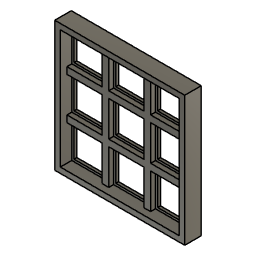
Master Assembly (Autodesk Fusion 360 archive; units mm, degrees)
design "Case Keys"
Autodesk Fusion 360 part; units mm, degrees
sketch "Sketch1" plane through (0, 0, 0) normal (0, 1, 0) x (1, 0, 0)
  line L0 (0, 0) -> (19.05, 0)
  line L1 (19.05, 0) -> (19.05, -19.05)
  line L2 (19.05, -19.05) -> (0, -19.05)
  line L3 (0, -19.05) -> (0, 0)
  line L4 (2.525, -2.525) -> (16.525, -2.525)
  line L5 (16.525, -2.525) -> (16.525, -16.525)
  line L6 (16.525, -16.525) -> (2.525, -16.525)
  line L7 (2.525, -16.525) -> (2.525, -2.525)
  line L8 (35.575, -16.525) -> (21.575, -16.525)
  line L9 (21.575, -2.525) -> (35.575, -2.525)
  line L10 (19.05, -19.05) -> (19.05, 0)
  line L11 (19.05, 0) -> (38.1, 0)
  line L12 (38.1, -19.05) -> (19.05, -19.05)
  line L13 (35.575, -2.525) -> (35.575, -16.525)
  line L14 (38.1, 0) -> (38.1, -19.05)
  line L15 (21.575, -16.525) -> (21.575, -2.525)
  line L16 (54.625, -16.525) -> (40.625, -16.525)
  line L17 (40.625, -2.525) -> (54.625, -2.525)
  line L18 (38.1, -19.05) -> (38.1, 0)
  line L19 (38.1, 0) -> (57.15, 0)
  line L20 (57.15, -19.05) -> (38.1, -19.05)
  line L21 (54.625, -2.525) -> (54.625, -16.525)
  line L22 (57.15, 0) -> (57.15, -19.05)
  line L23 (40.625, -16.525) -> (40.625, -2.525)
  line L24 (16.525, 2.525) -> (2.525, 2.525)
  line L25 (2.525, 16.525) -> (16.525, 16.525)
  line L26 (0, 0) -> (0, 19.05)
  line L27 (0, 19.05) -> (19.05, 19.05)
  line L28 (19.05, 0) -> (0, 0)
  line L29 (16.525, 16.525) -> (16.525, 2.525)
  line L30 (19.05, 19.05) -> (19.05, 0)
  line L31 (2.525, 2.525) -> (2.525, 16.525)
  line L32 (35.575, 2.525) -> (21.575, 2.525)
  line L33 (21.575, 16.525) -> (35.575, 16.525)
  line L34 (19.05, 0) -> (19.05, 19.05)
  line L35 (19.05, 19.05) -> (38.1, 19.05)
  line L36 (38.1, 0) -> (19.05, 0)
  line L37 (35.575, 16.525) -> (35.575, 2.525)
  line L38 (38.1, 19.05) -> (38.1, 0)
  line L39 (21.575, 2.525) -> (21.575, 16.525)
  line L40 (54.625, 2.525) -> (40.625, 2.525)
  line L41 (40.625, 16.525) -> (54.625, 16.525)
  line L42 (38.1, 0) -> (38.1, 19.05)
  line L43 (38.1, 19.05) -> (57.15, 19.05)
  line L44 (57.15, 0) -> (38.1, 0)
  line L45 (54.625, 16.525) -> (54.625, 2.525)
  line L46 (57.15, 19.05) -> (57.15, 0)
  line L47 (40.625, 2.525) -> (40.625, 16.525)
  line L48 (16.525, 21.575) -> (2.525, 21.575)
  line L49 (2.525, 35.575) -> (16.525, 35.575)
  line L50 (0, 19.05) -> (0, 38.1)
  line L51 (0, 38.1) -> (19.05, 38.1)
  line L52 (19.05, 19.05) -> (0, 19.05)
  line L53 (16.525, 35.575) -> (16.525, 21.575)
  line L54 (19.05, 38.1) -> (19.05, 19.05)
  line L55 (2.525, 21.575) -> (2.525, 35.575)
  line L56 (35.575, 21.575) -> (21.575, 21.575)
  line L57 (21.575, 35.575) -> (35.575, 35.575)
  line L58 (19.05, 19.05) -> (19.05, 38.1)
  line L59 (19.05, 38.1) -> (38.1, 38.1)
  line L60 (38.1, 19.05) -> (19.05, 19.05)
  line L61 (35.575, 35.575) -> (35.575, 21.575)
  line L62 (38.1, 38.1) -> (38.1, 19.05)
  line L63 (21.575, 21.575) -> (21.575, 35.575)
  line L64 (54.625, 21.575) -> (40.625, 21.575)
  line L65 (40.625, 35.575) -> (54.625, 35.575)
  line L66 (38.1, 19.05) -> (38.1, 38.1)
  line L67 (38.1, 38.1) -> (57.15, 38.1)
  line L68 (57.15, 19.05) -> (38.1, 19.05)
  line L69 (54.625, 35.575) -> (54.625, 21.575)
  line L70 (57.15, 38.1) -> (57.15, 19.05)
  line L71 (40.625, 21.575) -> (40.625, 35.575)
  circle A0 centre (9.525, -9.525) radius 1
  point P0 (19.05, 0)
  point P1 (38.1, 0)
  point P2 (0, 19.05)
  point P3 (19.05, 19.05)
  point P4 (38.1, 19.05)
  point P5 (0, 38.1)
  point P6 (19.05, 38.1)
  point P7 (38.1, 38.1)
  dimension "d13" = 19.05
  dimension "d14" = 19.05
  dimension "d15" = 2.525
  dimension "d18" = 38.1
  dimension "d19" = 38.1
  dimension "d41" = 2
  constraint horizontal L0
  constraint vertical L1
  constraint horizontal L2
  constraint vertical L3
  constraint coincident L0.start L3.end
  measures "d13" distance of L0.start L2.end
  measures "d14" distance of L0.start P0
  measures "d41" diameter of A0
extrude "Extrude1" add sketch "Sketch1" along normal blind 6.5 contours L0 L26 L27 L28 L30 L34 L52 | L0 L1 L2 L3 L10 L28 | L1 L10 L11 L12 L14 L18 L36 | L11 L30 L34 L35 L36 L38 L42 L60 | L27 L50 L51 L52 L54 L58 | L14 L18 L19 L20 L22 L44 | L19 L38 L42 L43 L44 L46 L68 | L35 L54 L58 L59 L60 L62 L66 | L43 L62 L66 L67 L68 L70
sketch "Sketch2" plane through (0, 0, 0) normal (0, 1, 0) x (1, 0, 0)
  line L0 (55.625, -17.525) -> (39.625, -17.525)
  line L1 (39.625, -17.525) -> (39.625, -1.525)
  line L2 (39.625, -1.525) -> (55.625, -1.525)
  line L3 (55.625, -1.525) -> (55.625, -17.525)
  line L4 (54.625, -16.525) -> (40.625, -16.525)
  line L5 (54.625, -2.525) -> (54.625, -16.525)
  line L6 (20.575, -1.525) -> (36.575, -1.525)
  line L7 (35.575, -2.525) -> (35.575, -16.525)
  line L8 (36.575, -1.525) -> (36.575, -17.525)
  line L9 (35.575, -16.525) -> (21.575, -16.525)
  line L10 (36.575, -17.525) -> (20.575, -17.525)
  line L11 (20.575, -17.525) -> (20.575, -1.525)
  line L12 (1.525, -1.525) -> (17.525, -1.525)
  line L13 (16.525, -2.525) -> (16.525, -16.525)
  line L14 (17.525, -1.525) -> (17.525, -17.525)
  line L15 (16.525, -16.525) -> (2.525, -16.525)
  line L16 (17.525, -17.525) -> (1.525, -17.525)
  line L17 (1.525, -17.525) -> (1.525, -1.525)
  line L18 (39.625, 17.525) -> (55.625, 17.525)
  line L19 (54.625, 16.525) -> (54.625, 2.525)
  line L20 (55.625, 17.525) -> (55.625, 1.525)
  line L21 (54.625, 2.525) -> (40.625, 2.525)
  line L22 (55.625, 1.525) -> (39.625, 1.525)
  line L23 (39.625, 1.525) -> (39.625, 17.525)
  line L24 (20.575, 17.525) -> (36.575, 17.525)
  line L25 (35.575, 16.525) -> (35.575, 2.525)
  line L26 (36.575, 17.525) -> (36.575, 1.525)
  line L27 (35.575, 2.525) -> (21.575, 2.525)
  line L28 (36.575, 1.525) -> (20.575, 1.525)
  line L29 (20.575, 1.525) -> (20.575, 17.525)
  line L30 (1.525, 17.525) -> (17.525, 17.525)
  line L31 (16.525, 16.525) -> (16.525, 2.525)
  line L32 (17.525, 17.525) -> (17.525, 1.525)
  line L33 (16.525, 2.525) -> (2.525, 2.525)
  line L34 (17.525, 1.525) -> (1.525, 1.525)
  line L35 (1.525, 1.525) -> (1.525, 17.525)
  line L36 (39.625, 36.575) -> (55.625, 36.575)
  line L37 (54.625, 35.575) -> (54.625, 21.575)
  line L38 (55.625, 36.575) -> (55.625, 20.575)
  line L39 (54.625, 21.575) -> (40.625, 21.575)
  line L40 (55.625, 20.575) -> (39.625, 20.575)
  line L41 (39.625, 20.575) -> (39.625, 36.575)
  line L42 (20.575, 36.575) -> (36.575, 36.575)
  line L43 (35.575, 35.575) -> (35.575, 21.575)
  line L44 (36.575, 36.575) -> (36.575, 20.575)
  line L45 (35.575, 21.575) -> (21.575, 21.575)
  line L46 (36.575, 20.575) -> (20.575, 20.575)
  line L47 (20.575, 20.575) -> (20.575, 36.575)
  line L48 (1.525, 36.575) -> (17.525, 36.575)
  line L49 (16.525, 35.575) -> (16.525, 21.575)
  line L50 (17.525, 36.575) -> (17.525, 20.575)
  line L51 (16.525, 21.575) -> (2.525, 21.575)
  line L52 (17.525, 20.575) -> (1.525, 20.575)
  line L53 (1.525, 20.575) -> (1.525, 36.575)
  dimension "d26" = 1
  dimension "d27" = 1
  dimension "d28" = 16
  dimension "d29" = 16
  dimension "d32" = -38.1
  dimension "d33" = 38.1
  constraint horizontal L0
  constraint vertical L1
  constraint horizontal L2
  constraint vertical L3
  measures "d26" distance of L0 L4
  measures "d27" distance of L3 L5
  measures "d28" distance of L0.start L0.end
  measures "d29" distance of L0.end L1.end
extrude "Extrude2" cut sketch "Sketch2" along normal blind 5.2
sketch "Sketch3" plane through (0, 6.5, 0) normal (0, 1, 0) x (-1, 0, 0)
  line L0 (-35.575, -21.575) -> (-21.575, -21.575)
  line L1 (-21.575, -21.575) -> (-21.575, -35.575)
  line L2 (-21.575, -35.575) -> (-35.575, -35.575)
  line L3 (-35.575, -35.575) -> (-35.575, -21.575)
  line L4 (-16.525, 16.525) -> (-2.525, 16.525)
  line L5 (-2.525, 16.525) -> (-2.525, 2.525)
  line L6 (-2.525, 2.525) -> (-16.525, 2.525)
  line L7 (-16.525, 2.525) -> (-16.525, 16.525)
  line L8 (-35.575, 16.525) -> (-21.575, 16.525)
  line L9 (-21.575, 16.525) -> (-21.575, 2.525)
  line L10 (-21.575, 2.525) -> (-35.575, 2.525)
  line L11 (-35.575, 2.525) -> (-35.575, 16.525)
  line L12 (-54.625, 16.525) -> (-40.625, 16.525)
  line L13 (-40.625, 16.525) -> (-40.625, 2.525)
  line L14 (-40.625, 2.525) -> (-54.625, 2.525)
  line L15 (-54.625, 2.525) -> (-54.625, 16.525)
  line L16 (-35.575, -2.525) -> (-21.575, -2.525)
  line L17 (-21.575, -2.525) -> (-21.575, -16.525)
  line L18 (-21.575, -16.525) -> (-35.575, -16.525)
  line L19 (-35.575, -16.525) -> (-35.575, -2.525)
  line L20 (-54.625, -21.575) -> (-40.625, -21.575)
  line L21 (-40.625, -21.575) -> (-40.625, -35.575)
  line L22 (-40.625, -35.575) -> (-54.625, -35.575)
  line L23 (-54.625, -35.575) -> (-54.625, -21.575)
  line L24 (-54.625, -2.525) -> (-40.625, -2.525)
  line L25 (-40.625, -2.525) -> (-40.625, -16.525)
  line L26 (-40.625, -16.525) -> (-54.625, -16.525)
  line L27 (-54.625, -16.525) -> (-54.625, -2.525)
  line L28 (-16.525, -2.525) -> (-2.525, -2.525)
  line L29 (-2.525, -2.525) -> (-2.525, -16.525)
  line L30 (-2.525, -16.525) -> (-16.525, -16.525)
  line L31 (-16.525, -16.525) -> (-16.525, -2.525)
  line L32 (-16.525, -21.575) -> (-2.525, -21.575)
  line L33 (-2.525, -21.575) -> (-2.525, -35.575)
  line L34 (-2.525, -35.575) -> (-16.525, -35.575)
  line L35 (-16.525, -35.575) -> (-16.525, -21.575)
  line L36 (-57.15, -38.1) -> (0, -38.1)
  line L37 (0, -38.1) -> (0, 19.05)
  line L38 (0, 19.05) -> (-57.15, 19.05)
  line L39 (-57.15, 19.05) -> (-57.15, -38.1)
  line L40 (1, 20.05) -> (-58.15, 20.05)
  line L41 (-58.15, 20.05) -> (-58.15, -39.1)
  line L42 (-58.15, -39.1) -> (1, -39.1)
  line L43 (1, -39.1) -> (1, 20.05)
  dimension "d36" = 1
extrude "Extrude3" add sketch "Sketch3" along normal blind 1 and the other way up to surface (6.5 mm away) contours L40 L41 L42 L43
sketch "Sketch4" plane through (0, 0, 0) normal (0, -1, 0) x (1, 0, 0)
  line L0 (58.15, 20.05) -> (-1, 20.05)
  line L1 (-1, 20.05) -> (-1, -39.1)
  line L2 (-1, -39.1) -> (58.15, -39.1)
  line L3 (58.15, -39.1) -> (58.15, 20.05)
  line L4 (1.525, 1.525) -> (1.525, 17.525)
  line L5 (1.525, 17.525) -> (17.525, 17.525)
  line L6 (17.525, 17.525) -> (17.525, 1.525)
  line L7 (17.525, 1.525) -> (1.525, 1.525)
  line L8 (39.625, -36.575) -> (39.625, -20.575)
  line L9 (39.625, -20.575) -> (55.625, -20.575)
  line L10 (55.625, -20.575) -> (55.625, -36.575)
  line L11 (55.625, -36.575) -> (39.625, -36.575)
  line L12 (39.625, -17.525) -> (39.625, -1.525)
  line L13 (39.625, -1.525) -> (55.625, -1.525)
  line L14 (55.625, -1.525) -> (55.625, -17.525)
  line L15 (55.625, -17.525) -> (39.625, -17.525)
  line L16 (20.575, -36.575) -> (20.575, -20.575)
  line L17 (20.575, -20.575) -> (36.575, -20.575)
  line L18 (36.575, -20.575) -> (36.575, -36.575)
  line L19 (36.575, -36.575) -> (20.575, -36.575)
  line L20 (1.525, -17.525) -> (1.525, -1.525)
  line L21 (1.525, -1.525) -> (17.525, -1.525)
  line L22 (17.525, -1.525) -> (17.525, -17.525)
  line L23 (17.525, -17.525) -> (1.525, -17.525)
  line L24 (20.575, 1.525) -> (20.575, 17.525)
  line L25 (20.575, 17.525) -> (36.575, 17.525)
  line L26 (36.575, 17.525) -> (36.575, 1.525)
  line L27 (36.575, 1.525) -> (20.575, 1.525)
  line L28 (55.625, 17.525) -> (55.625, 1.525)
  line L29 (55.625, 1.525) -> (39.625, 1.525)
  line L30 (39.625, 1.525) -> (39.625, 17.525)
  line L31 (39.625, 17.525) -> (55.625, 17.525)
  line L32 (20.575, -17.525) -> (20.575, -1.525)
  line L33 (20.575, -1.525) -> (36.575, -1.525)
  line L34 (36.575, -1.525) -> (36.575, -17.525)
  line L35 (36.575, -17.525) -> (20.575, -17.525)
  line L36 (1.525, -36.575) -> (1.525, -20.575)
  line L37 (1.525, -20.575) -> (17.525, -20.575)
  line L38 (17.525, -20.575) -> (17.525, -36.575)
  line L39 (17.525, -36.575) -> (1.525, -36.575)
  line L40 (1.525, 17.525) -> (55.625, 17.525)
  line L41 (55.625, 17.525) -> (55.625, -36.575)
  line L42 (55.625, -36.575) -> (1.525, -36.575)
  line L43 (1.525, -36.575) -> (1.525, 17.525)
  constraint horizontal L40
  constraint vertical L41
  constraint horizontal L42
  constraint vertical L43
  constraint coincident L10.end L11.start
  constraint coincident L4.end L5.start
extrude "Extrude4" cut sketch "Sketch4" against normal blind 3 contours L4 L5 L6 L7 L40 L43 | L6 L7 L8 L9 L12 L13 L15 L16 L17 L18 L21 L22 L23 L24 L26 L27 L29 L30 L37 L38 L40 L41 L42 L43 | L20 L21 L22 L23 L43 | L24 L25 L26 L27 L40 | L36 L37 L38 L39 L42 L43 | L28 L29 L30 L31 L40 L41 | L16 L17 L18 L19 L42 | L12 L13 L14 L15 L41 | L8 L9 L10 L11 L41 L42 | L32 L33 L34 L35
